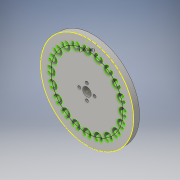
# Autodesk Inventor part: Ball Launcher Wheel
Saved by Autodesk Inventor 2016 SP2 (Build 200236200, 236)
## iProperties
Created: 2017-01-18
Part Number: Ball Launcher Wheel
Material: Generic
Document SubType Name: Modeling
Designer: 17hibdont0103
Density: 1 g/cm^3
Appearance: Default
Author: 17hibdont0103
Autodesk Inventor part; units mm, degrees
ref_plane "YZ Plane" through (0, 0, 0) normal (1, 0, 0) x (0, 1, 0)
ref_plane "XZ Plane" through (0, 0, 0) normal (0, 1, 0) x (-1, 0, 0)
ref_plane "XY Plane" through (0, 0, 0) normal (0, 0, 1) x (1, 0, 0)
sketch "Sketch1" plane through (0, 0, 0) normal (0, 0, 1) x (1, 0, 0)
  circle A0 centre (0, 0) radius 48.8061
  circle A1 centre (0, 0) radius 4.4958
  circle A2 centre (0, 8.001) radius 1.5875
  circle A3 centre (-8.001, 0) radius 1.5875
  circle A4 centre (0, -8.001) radius 1.5875
  circle A5 centre (8.001, 0) radius 1.5875
  dimension "d0" = 97.6122
  dimension "d1" = 8.9916
  dimension "d3" = 3.175
  dimension "d6" = 360
  constraints: 6 centre point, 2 coincident, 9 other
  measures "d0" diameter of A0
  measures "d1" diameter of A1
  measures "d3" diameter of A2
extrude "Extrusion1" add sketch "Sketch1" along normal blind 6.35
sketch "Sketch2" plane through (0, 0, 6.35) normal (0, 0, 1) x (1, 0, 0)
  circle A0 centre (0, 0) radius 48.8061 projected
  arc A1 (-1.1716, 39.3079) -> (1.1716, 39.3079) centre (0, 37.7063) ccw
  arc A2 (-2.9818, 41.4198) -> (3.2192, 41.216) centre (0, 37.7063) ccw
  arc A3 (-1.1716, 39.3079) -> (-2.9818, 41.4198) centre (-2.4693, 40.0273) ccw
  arc A4 (3.2192, 41.216) -> (1.1716, 39.3079) centre (2.5148, 39.9192) ccw
  arc A5 (-15.6353, 38.4711) -> (-9.6748, 40.1936) centre (-11.6519, 35.8608) ccw
  arc A6 (-13.261, 37.022) -> (-11.0326, 37.7461) centre (-11.6519, 35.8608) ccw
  arc A7 (-9.6748, 40.1936) -> (-11.0326, 37.7461) centre (-9.944, 38.7425) ccw
  arc A8 (-13.261, 37.022) -> (-15.6353, 38.4711) centre (-14.7176, 37.3052) ccw
  arc A9 (-26.7583, 31.7566) -> (-21.6218, 35.2367) centre (-22.1632, 30.505) ccw
  arc A10 (-24.0524, 31.1121) -> (-22.1568, 32.4894) centre (-22.1632, 30.505) ccw
  arc A11 (-21.6218, 35.2367) -> (-22.1568, 32.4894) centre (-21.4294, 33.7735) ccw
  arc A12 (-24.0524, 31.1121) -> (-26.7583, 31.7566) centre (-25.5252, 30.9314) ccw
  arc A13 (-35.262, 21.9336) -> (-31.4523, 26.8306) centre (-30.505, 22.1632) ccw
  arc A14 (-32.4894, 22.1568) -> (-31.1121, 24.0524) centre (-30.505, 22.1632) ccw
  arc A15 (-31.4523, 26.8306) -> (-31.1121, 24.0524) centre (-30.8171, 25.4984) ccw
  arc A16 (-32.4894, 22.1568) -> (-35.262, 21.9336) centre (-33.8342, 21.5298) ccw
  arc A17 (-40.314, 9.9635) -> (-38.204, 15.7981) centre (-35.8608, 11.6519) ccw
  arc A18 (-37.7461, 11.0326) -> (-37.022, 13.261) centre (-35.8608, 11.6519) ccw
  arc A19 (-38.204, 15.7981) -> (-37.022, 13.261) centre (-37.1883, 14.7274) ccw
  arc A20 (-37.7461, 11.0326) -> (-40.314, 9.9635) centre (-38.8313, 10.0207) ccw
  arc A21 (-41.4198, -2.9818) -> (-41.216, 3.2192) centre (-37.7063, 0) ccw
  arc A22 (-39.3079, -1.1716) -> (-39.3079, 1.1716) centre (-37.7063, 0) ccw
  arc A23 (-41.216, 3.2192) -> (-39.3079, 1.1716) centre (-39.9192, 2.5148) ccw
  arc A24 (-39.3079, -1.1716) -> (-41.4198, -2.9818) centre (-40.0273, -2.4693) ccw
  arc A25 (-38.4711, -15.6353) -> (-40.1936, -9.6748) centre (-35.8608, -11.6519) ccw
  arc A26 (-37.022, -13.261) -> (-37.7461, -11.0326) centre (-35.8608, -11.6519) ccw
  arc A27 (-40.1936, -9.6748) -> (-37.7461, -11.0326) centre (-38.7425, -9.944) ccw
  arc A28 (-37.022, -13.261) -> (-38.4711, -15.6353) centre (-37.3052, -14.7176) ccw
  arc A29 (-31.7566, -26.7583) -> (-35.2367, -21.6218) centre (-30.505, -22.1632) ccw
  arc A30 (-31.1121, -24.0524) -> (-32.4894, -22.1568) centre (-30.505, -22.1632) ccw
  arc A31 (-35.2367, -21.6218) -> (-32.4894, -22.1568) centre (-33.7735, -21.4294) ccw
  arc A32 (-31.1121, -24.0524) -> (-31.7566, -26.7583) centre (-30.9314, -25.5252) ccw
  arc A33 (-21.9336, -35.262) -> (-26.8306, -31.4523) centre (-22.1632, -30.505) ccw
  arc A34 (-22.1568, -32.4894) -> (-24.0524, -31.1121) centre (-22.1632, -30.505) ccw
  arc A35 (-26.8306, -31.4523) -> (-24.0524, -31.1121) centre (-25.4984, -30.8171) ccw
  arc A36 (-22.1568, -32.4894) -> (-21.9336, -35.262) centre (-21.5298, -33.8342) ccw
  arc A37 (-9.9635, -40.314) -> (-15.7981, -38.204) centre (-11.6519, -35.8608) ccw
  arc A38 (-11.0326, -37.7461) -> (-13.261, -37.022) centre (-11.6519, -35.8608) ccw
  arc A39 (-15.7981, -38.204) -> (-13.261, -37.022) centre (-14.7274, -37.1883) ccw
  arc A40 (-11.0326, -37.7461) -> (-9.9635, -40.314) centre (-10.0207, -38.8313) ccw
  arc A41 (2.9818, -41.4198) -> (-3.2192, -41.216) centre (0, -37.7063) ccw
  arc A42 (1.1716, -39.3079) -> (-1.1716, -39.3079) centre (0, -37.7063) ccw
  arc A43 (-3.2192, -41.216) -> (-1.1716, -39.3079) centre (-2.5148, -39.9192) ccw
  arc A44 (1.1716, -39.3079) -> (2.9818, -41.4198) centre (2.4693, -40.0273) ccw
  arc A45 (15.6353, -38.4711) -> (9.6748, -40.1936) centre (11.6519, -35.8608) ccw
  arc A46 (13.261, -37.022) -> (11.0326, -37.7461) centre (11.6519, -35.8608) ccw
  arc A47 (9.6748, -40.1936) -> (11.0326, -37.7461) centre (9.944, -38.7425) ccw
  arc A48 (13.261, -37.022) -> (15.6353, -38.4711) centre (14.7176, -37.3052) ccw
  arc A49 (26.7583, -31.7566) -> (21.6218, -35.2367) centre (22.1632, -30.505) ccw
  arc A50 (24.0524, -31.1121) -> (22.1568, -32.4894) centre (22.1632, -30.505) ccw
  arc A51 (21.6218, -35.2367) -> (22.1568, -32.4894) centre (21.4294, -33.7735) ccw
  arc A52 (24.0524, -31.1121) -> (26.7583, -31.7566) centre (25.5252, -30.9314) ccw
  arc A53 (35.262, -21.9336) -> (31.4523, -26.8306) centre (30.505, -22.1632) ccw
  arc A54 (32.4894, -22.1568) -> (31.1121, -24.0524) centre (30.505, -22.1632) ccw
  arc A55 (31.4523, -26.8306) -> (31.1121, -24.0524) centre (30.8171, -25.4984) ccw
  arc A56 (32.4894, -22.1568) -> (35.262, -21.9336) centre (33.8342, -21.5298) ccw
  arc A57 (40.314, -9.9635) -> (38.204, -15.7981) centre (35.8608, -11.6519) ccw
  arc A58 (37.7461, -11.0326) -> (37.022, -13.261) centre (35.8608, -11.6519) ccw
  arc A59 (38.204, -15.7981) -> (37.022, -13.261) centre (37.1883, -14.7274) ccw
  arc A60 (37.7461, -11.0326) -> (40.314, -9.9635) centre (38.8313, -10.0207) ccw
  arc A61 (41.4198, 2.9818) -> (41.216, -3.2192) centre (37.7063, 0) ccw
  arc A62 (39.3079, 1.1716) -> (39.3079, -1.1716) centre (37.7063, 0) ccw
  arc A63 (41.216, -3.2192) -> (39.3079, -1.1716) centre (39.9192, -2.5148) ccw
  arc A64 (39.3079, 1.1716) -> (41.4198, 2.9818) centre (40.0273, 2.4693) ccw
  arc A65 (38.4711, 15.6353) -> (40.1936, 9.6748) centre (35.8608, 11.6519) ccw
  arc A66 (37.022, 13.261) -> (37.7461, 11.0326) centre (35.8608, 11.6519) ccw
  arc A67 (40.1936, 9.6748) -> (37.7461, 11.0326) centre (38.7425, 9.944) ccw
  arc A68 (37.022, 13.261) -> (38.4711, 15.6353) centre (37.3052, 14.7176) ccw
  arc A69 (31.7566, 26.7583) -> (35.2367, 21.6218) centre (30.505, 22.1632) ccw
  arc A70 (31.1121, 24.0524) -> (32.4894, 22.1568) centre (30.505, 22.1632) ccw
  arc A71 (35.2367, 21.6218) -> (32.4894, 22.1568) centre (33.7735, 21.4294) ccw
  arc A72 (31.1121, 24.0524) -> (31.7566, 26.7583) centre (30.9314, 25.5252) ccw
  arc A73 (21.9336, 35.262) -> (26.8306, 31.4523) centre (22.1632, 30.505) ccw
  arc A74 (22.1568, 32.4894) -> (24.0524, 31.1121) centre (22.1632, 30.505) ccw
  arc A75 (26.8306, 31.4523) -> (24.0524, 31.1121) centre (25.4984, 30.8171) ccw
  arc A76 (22.1568, 32.4894) -> (21.9336, 35.262) centre (21.5298, 33.8342) ccw
  arc A77 (9.9635, 40.314) -> (15.7981, 38.204) centre (11.6519, 35.8608) ccw
  arc A78 (11.0326, 37.7461) -> (13.261, 37.022) centre (11.6519, 35.8608) ccw
  arc A79 (15.7981, 38.204) -> (13.261, 37.022) centre (14.7274, 37.1883) ccw
  arc A80 (11.0326, 37.7461) -> (9.9635, 40.314) centre (10.0207, 38.8313) ccw
  point P0 (0, 45.9646)
  dimension "d38" = 360
  constraints: 160 point on circle, 80 centre point, 20 coincident, 241 other
extrude "Extrusion2" [suppressed]
extrude "Extrusion3" cut sketch "Sketch2" against normal blind 6.35 keep common part
body "Solid1"
